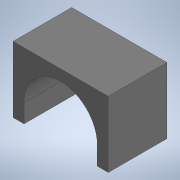
# Autodesk Inventor part: shadeHolder
Saved by Autodesk Inventor 2021.2 (Build 252289000, 289)
## iProperties
Created: 2021-02-12
Part Number: shadeHolder
Material: PC/ABS Plastic
Document SubType Name: Modeling
Designer: robst
Density: 0.357273 g/cm^3
Appearance: Gray
Author: robst
Autodesk Inventor part; units mm, degrees
ref_plane "YZ Plane" through (0, 0, 0) normal (1, 0, 0) x (0, 1, 0)
ref_plane "XZ Plane" through (0, 0, 0) normal (0, 1, 0) x (-1, 0, 0)
ref_plane "XY Plane" through (0, 0, 0) normal (0, 0, 1) x (1, 0, 0)
sketch "Sketch1" plane through (0, 0, 0) normal (0, 0, 1) x (1, 0, 0)
  line L0 (0, -3.175) -> (0, 3.175) construction
  line L1 (6.35, 0) -> (6.35, 3.175)
  line L2 (-6.35, 3.175) -> (-6.35, 0)
  arc A0 (6.35, 3.175) -> (-6.35, 3.175) centre (0, 3.175) ccw
  line L3 (8.255, 0) -> (8.255, 11.43)
  line L4 (8.255, 11.43) -> (-8.255, 11.43)
  line L5 (-8.255, 11.43) -> (-8.255, 0)
  line L6 (-8.255, -11.43) -> (8.255, 11.43) construction
  line L7 (8.255, -11.43) -> (-8.255, 11.43) construction
  line L8 (8.255, 0) -> (6.35, 0)
  line L9 (-6.35, 0) -> (-8.255, 0)
  point P0 (0, 0)
  point P1 (-5.062, -7.0089)
  dimension "d0" = 6.35
  dimension "d3" = 1.905
  constraints: 22 end point, 3 midpoint, 2 parallel, 2 point on circle, 2 tangent, 1 centre point, 1 point on line, 1 vertical
  measures "d0" radius of A0
  measures "d3" distance between parallel lines of L3 L1
extrude "Extrusion3" add sketch "Sketch1" along normal mid plane 10.16
body "Solid1"
body "Solid2"
